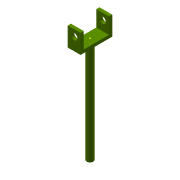
# Autodesk Inventor part: PC3.5-ROD
Saved by Autodesk Inventor 2015 (Build 190159000, 159)
## iProperties
Created: 2015-01-13
Part Number: PC3.5-ROD
Material: Generic
Document SubType Name: Modeling
Designer: Collin_2
Density: 1 g/cm^3
Appearance: Default
Author: Collin_2
Autodesk Inventor part; units mm, degrees
ref_plane "YZ Plane" through (0, 0, 0) normal (1, 0, 0) x (0, 1, 0)
ref_plane "XZ Plane" through (0, 0, 0) normal (0, 1, 0) x (-1, 0, 0)
ref_plane "XY Plane" through (0, 0, 0) normal (0, 0, 1) x (1, 0, 0)
sketch "Sketch1" plane through (0, 0, 0) normal (0, 1, 0) x (-1, 0, 0)
  circle A0 centre (0, 0) radius 3.175
  dimension "d0" = 6.35
  constraints: 1 centre point, 1 coincident
  measures "d0" diameter of A0
extrude "Extrusion1" add sketch "Sketch1" along normal blind 101.6
sketch "Sketch2" plane through (0, 101.6, 0) normal (0, 1, 0) x (1, 0, 0)
  line L0 (6.35, -15.748) -> (-6.35, -15.748)
  line L1 (-6.35, -15.748) -> (-6.35, 15.748)
  line L2 (-6.35, 15.748) -> (6.35, 15.748)
  line L3 (6.35, 15.748) -> (6.35, -15.748)
  line L4 (6.35, -15.748) -> (-6.35, 15.748) construction
  line L5 (-6.35, -15.748) -> (6.35, 15.748) construction
  point P0 (0, 0)
  dimension "d3" = 12.7
  dimension "d4" = 31.496
  constraints: 12 end point, 2 midpoint, 2 parallel, 1 horizontal, 1 perpendicular
  measures "d3" distance of L1.end L2.end
  measures "d4" distance of L0.end L1.end
extrude "Extrusion2" add sketch "Sketch2" along normal blind 3.175
sketch "Sketch3" plane through (0, 104.775, 0) normal (0, 1, 0) x (1, 0, 0)
  point P0 (0, 0)
sketch "Sketch4" plane through (0, 104.775, 0) normal (0, 1, 0) x (1, 0, 0)
  line L0 (6.35, -15.748) -> (6.35, 15.748) projected
  line L1 (-6.35, -15.748) -> (6.35, -15.748)
  line L2 (6.35, -15.748) -> (6.35, -12.573)
  line L3 (6.35, -12.573) -> (-6.35, -12.573)
  line L4 (-6.35, -12.573) -> (-6.35, -15.748)
  line L5 (-6.35, 15.748) -> (6.35, 15.748)
  line L6 (6.35, 15.748) -> (6.35, 12.573)
  line L7 (6.35, 12.573) -> (-6.35, 12.573)
  line L8 (-6.35, 12.573) -> (-6.35, 15.748)
  line L9 (6.35, 15.748) -> (-6.35, 15.748) projected
  point P0 (0, 0)
  dimension "d7" = 3.175
  dimension "d8" = 3.175
  dimension "d9" = 0
  constraints: 16 end point, 4 parallel, 2 horizontal, 2 perpendicular, 2 point on line
  measures "d7" distance of L3.end L1.start
  measures "d8" distance of L7.end L5.start
  measures "d9" distance between parallel lines of L5 L9
extrude "Extrusion3" add sketch "Sketch4" along normal blind 15.875
sketch "Sketch5" plane through (6.35, 101.6, -15.748) normal (0, 0, -1) x (-1, 0, 0)
  circle A0 centre (6.35, 12.7) radius 3.175
  line L0 (12.7, 0) -> (0, 0) projected
  point P0 (6.35, -101.6)
  dimension "d12" = 6.35
  dimension "d13" = 12.7
  constraints: 1 centre point
  measures "d12" diameter of A0
  measures "d13" distance from line of L0 A0.centre
extrude "Extrusion4" cut sketch "Sketch5" against normal blind 50.8
body "Solid1"
